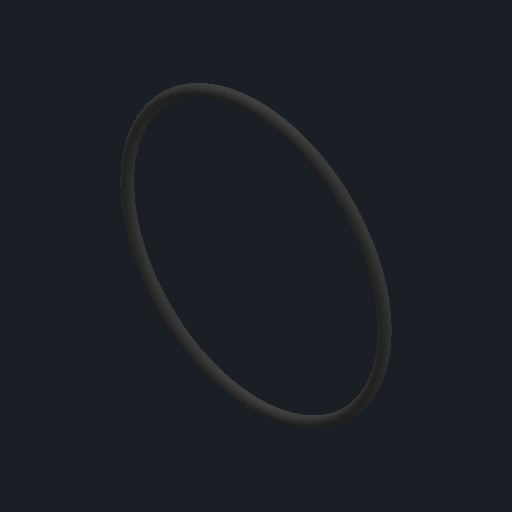
# Autodesk Inventor part: oring-102-110
Saved by Autodesk Inventor 2026 (Build 300175050, 175E)
## iProperties
Created: 2025-12-11
Part Number: oring-102-110
Material: Rubber, Silicone
Document SubType Name: Modeling
Designer: queezz
Density: 1.25 g/cm^3
Appearance: Rubber - Black
Author: queezz
Autodesk Inventor part; units mm, degrees
ref_plane "YZ Plane" through (0, 0, 0) normal (1, 0, 0) x (0, 1, 0)
ref_plane "XZ Plane" through (0, 0, 0) normal (0, 1, 0) x (-1, 0, 0)
ref_plane "XY Plane" through (0, 0, 0) normal (0, 0, 1) x (1, 0, 0)
sketch "Sketch1" plane through (0, 0, 0) normal (0, 1, 0) x (-1, 0, 0)
  line L0 (0, 5.4773) -> (0, 0)
  circle A0 centre (53, 0) radius 2
  dimension "d0" = 4
  dimension "d1" = 106
  constraints: 2 end point, 1 centre point, 1 vertical
  measures "d0" diameter of A0
  measures "d1" diameter of A0.centre L0
revolve "Revolution1" add sketch "Sketch1" angle 360 about axis through (0, 0, 5.4773) along (0, 0, -1)
body "Solid1"
